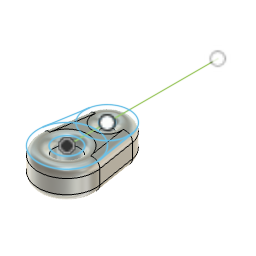
mmono (Autodesk Fusion 360 design; units mm, degrees)
Autodesk Fusion 360 part; units mm, degrees
sketch "Sketch1" plane through (0, 0, 0) normal (0, 0, 1) x (1, 0, 0)
  line L0 (0, -0.0218) -> (0, 150)
  circle A0 centre (0, -0.0218) radius 12.5
  circle A1 centre (0, -0.0218) radius 28.5
  circle A2 centre (0.0333, 39.9782) radius 6
  circle A3 centre (0.0333, 39.9782) radius 22
  line L1 (21.7439, 43.5351) -> (28.125, 4.586)
  line L2 (-21.6713, 43.5713) -> (-28.1173, 4.6329)
  dimension "d38" = 16
  dimension "d39" = 25
  dimension "d40" = 12
  dimension "d42" = 40
  dimension "d43" = 16
  constraint coincident L0.start A0.centre
  constraint coincident A3 L1.start
  constraint tangent A3 L1
  constraint coincident A1 L1.end
  constraint tangent A1 L1
  constraint coincident A3 L2.start
  constraint tangent A3 L2
  constraint coincident A1 L2.end
  constraint tangent A1 L2
  measures "d39" diameter of A0
  measures "d40" diameter of A2
  measures "d42" distance of L0.start A2.centre
extrude "Extrude6" add sketch "Sketch1" against normal blind 30 contours L0 A1 A3 | A1 A3 | L0 A1 A3 | L0 A1 A2 A3 | L0 A1 A2 A3 | A1 A3 L2 | A1 A3 L1 | A0
extrude "Extrude7" cut sketch "Sketch1" against normal blind 22.3431 contours A0
fillet "Fillet2" radius 8 1 edges at (-11.6541, 4.4984, 0)
fillet "Fillet2" radius 8 2 edges at (-5.5606, 42.1479, 0) (-5.5606, 37.8085, -30)
fillet "Fillet2" radius 8 8 edges at (-0.0237, -28.5218, 0) (24.9345, 24.0605, 0) (0.0517, 61.9782, 0) (-24.8943, 24.1021, 0) (-24.8943, 24.1021, -30) (0.0517, 61.9782, -30) (24.9345, 24.0605, -30) (-0.0237, -28.5218, -30)
